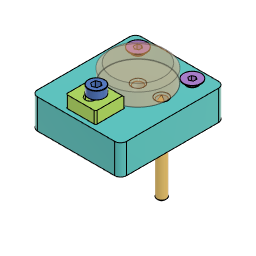
ChannelScoringJig_Parametric (Autodesk Fusion 360 design; units mm, degrees)
Autodesk Fusion 360 part; units mm, degrees
sketch "Sketch1" plane through (0, 0, 0) normal (0, 0, 1) x (1, 0, 0)
  line L0 (15, 17.5) -> (-15, 17.5)
  line L1 (-15, 17.5) -> (-15, -17.5)
  line L2 (-15, -17.5) -> (15, -17.5)
  line L3 (15, -17.5) -> (15, 17.5)
  line L4 (15, 17.5) -> (-15, -17.5) construction
  line L5 (-15, 17.5) -> (15, -17.5) construction
  dimension "d1" = 30
  dimension "d2" = 35
  constraint horizontal L0
  constraint perpendicular L0 L1
  constraint parallel L0 L2
  constraint parallel L1 L3
  constraint coincident L4 origin
  constraint coincident L5 origin
  measures "d1" distance of L0.start L0.end
  measures "d2" distance of L0.end L1.end
extrude "Extrude1" add sketch "Sketch1" along normal blind 10 makes body 1
sketch "Sketch2" plane through (0, 0, 10) normal (0, 0, 1) x (-1, 0, 0)
  line L0 (-15, 17.5) -> (-15, -17.5)
  line L1 (-15, -17.5) -> (15, -17.5)
  line L2 (15, -17.5) -> (15, 17.5)
  line L3 (15, 17.5) -> (-15, 17.5)
  circle A0 centre (9.157, -12.5) radius 1.35
  circle A1 centre (-9.157, -12.5) radius 1.35
  line L4 (9.157, -12.5) -> (-9.157, -12.5) construction
  line L5 (0, -12.5) -> (0, 0) construction
  circle A2 centre (0, -3.343) radius 12.95 construction
  line L6 (9.157, -12.5) -> (0, -3.343) construction
  line L7 (0, -3.343) -> (-9.157, -12.5) construction
  dimension "d5" = 2.7
  dimension "d42" = 5
  dimension "d67" = 25.9
  dimension "d70" = 90
  constraint coincident A0.centre L4.start
  constraint coincident A1.centre L4.end
  constraint horizontal L4
  constraint midpoint L4 L5.start
  constraint coincident L5.end origin
  constraint vertical L5
  constraint equal A0 A1
  constraint coincident L5 A2.centre
  constraint coincident A1.centre A2
  constraint coincident A2.centre L6.end
  measures "d5" diameter of A0
  measures "d42" distance of L1 L4
  measures "d67" diameter of A2
  measures "d70" angle of L6 L7
extrude "Extrude2" cut sketch "Sketch2" against normal blind 11 contours A0 | A1 bodies 1
sketch "Sketch3" plane through (0, 0, 10) normal (0, 0, 1) x (-1, 0, 0)
  line L0 (-15, 17.5) -> (-15, -17.5)
  line L1 (-15, -17.5) -> (15, -17.5)
  line L2 (15, -17.5) -> (15, 17.5)
  line L3 (15, 17.5) -> (-15, 17.5)
  circle A0 centre (0, -3.343) radius 10 construction
  circle A1 centre (9.157, -12.5) radius 2.95 construction
  circle A2 centre (0, -3.343) radius 1.6
  circle A3 centre (-8, -3.343) radius 1.6
  circle A4 centre (9.157, -12.5) radius 1.35
  point P0 (0, -13.343)
  point P1 (-10, -3.343)
  dimension "d10" = 20
  dimension "d11" = 5.9
  dimension "d12" = 3.2
  dimension "d13" = 3.2
  dimension "d53" = 2
  constraint tangent A0 A1
  constraint vertical origin A0.centre
  constraint concentric A1 A4
  constraint concentric A0 A2
  constraint coincident A0 P0
  constraint horizontal A0.centre A3.centre
  constraint coincident A0 P1
  constraint horizontal A0.centre P1
  measures "d10" diameter of A0
  measures "d11" diameter of A1
  measures "d12" diameter of A2
  measures "d13" diameter of A3
  measures "d53" distance of A3.centre P1
extrude "Extrude5" cut sketch "Sketch3" against normal blind 15 contours A2 | A3 bodies 1
sketch "Sketch6" plane through (0, 17.5, 0) normal (0, 1, 0) x (-1, 0, 0)
  line L0 (-15, 0) -> (15, 0)
  line L1 (15, 0) -> (15, 10)
  line L2 (15, 10) -> (-15, 10)
  line L3 (-15, 10) -> (-15, 0)
  line L4 (-4, 0) -> (-12, 0)
  line L5 (-12, 0) -> (-12, 3)
  line L6 (-9, 6) -> (-7, 6)
  line L7 (-4, 3) -> (-4, 0)
  arc A0 (-4, 3) -> (-7, 6) centre (-7, 3) ccw
  arc A1 (-9, 6) -> (-12, 3) centre (-9, 3) ccw
  dimension "d48" = 3
  dimension "d49" = 3
  dimension "d56" = 3
  dimension "d57" = 8
  constraint horizontal L4
  constraint vertical L5
  constraint horizontal L6
  constraint vertical L7
  constraint coincident L0 L4.start
  constraint tangent L6 A0
  constraint tangent L7 A0
  constraint tangent L5 A1
  constraint tangent L6 A1
  measures "d48" radius of A0
  measures "d49" radius of A1
  measures "d56" distance of L3 L5
  measures "d57" distance of L4.start L4.end
extrude "Extrude7" cut sketch "Sketch6" against normal blind 8.925 contours L0 L4 L5 L6 L7 A0 A1 bodies 1
sketch "Sketch10" plane through (0, 8.575, 0) normal (0, 1, 0) x (-1, 0, 0)
  arc A0 (-4, 3) -> (-7, 6) centre (-7, 3) ccw
  line L0 (-12, 0) -> (-4, 0)
  line L1 (-4, 0) -> (-4, 3)
  circle A1 centre (-8, 3) radius 1.35
  arc A2 (-9, 6) -> (-12, 3) centre (-9, 3) ccw
  line L2 (-12, 3) -> (-12, 0)
  line L3 (-7, 6) -> (-9, 6)
  dimension "d62" = 2.7
  dimension "d63" = 3
  dimension "d64" = 8
  measures "d62" diameter of A1
  measures "d63" distance of L0 A1.centre
  measures "d64" horizontal distance of origin A1.centre
extrude "Extrude10" cut sketch "Sketch10" along normal up to surface contours A1 end surface at (6.408, 3.5023, 6.6667) on bodies 1 bodies 1
fillet "Fillet2" radius 2 4 edges at (15, 17.5, 5) (-15, 17.5, 5) (15, -17.5, 5) (-15, -17.5, 5) on bodies 1
sketch "Sketch7" plane through (0, 0, 10) normal (0, 0, 1) x (-1, 0, 0)
  arc A0 (15, 15.5) -> (13, 17.5) centre (13, 15.5) ccw
  line L0 (13, 17.5) -> (-13, 17.5)
  arc A1 (-13, 17.5) -> (-15, 15.5) centre (-13, 15.5) ccw
  line L1 (-15, 15.5) -> (-15, -15.5)
  line L2 (15, -15.5) -> (15, 15.5)
  circle A2 centre (0, 10.657) radius 1.35
  circle A3 centre (0, -3.343) radius 1.6
  arc A4 (-15, -15.5) -> (-13, -17.5) centre (-13, -15.5) ccw
  line L3 (-13, -17.5) -> (13, -17.5)
  arc A5 (13, -17.5) -> (15, -15.5) centre (13, -15.5) ccw
  circle A6 centre (9.157, -12.5) radius 1.35
  circle A7 centre (-9.157, -12.5) radius 1.35
  circle A8 centre (-8, -3.343) radius 1.6
  dimension "d36" = 2.7
  dimension "d126" = 14
  constraint vertical origin A2.centre
  measures "d36" diameter of A2
  measures "d126" distance of A2.centre A3.centre
extrude "Extrude8" cut sketch "Sketch7" against normal blind 38 contours A2 bodies 1
chamfer "Chamfer1" distance 0.5 angle 45 9 edges at (9.4917, 3.9216, 0) (1.2586, -10.1689, 0) (-7.8984, 12.9882, 0) (-7.8984, 12.0118, 10) (10.4157, 12.0118, 10) (9.4917, 2.7644, 10) (1.2586, -11.1452, 10) (1.4917, 2.7644, 10) (1.4917, 3.9216, 0) on bodies 1
chamfer "Chamfer3" distance 0.5 angle 45 2 edges at (4, 13.0375, 0) (12, 13.0375, 0) measured on face at (8.4117, -8.1054, 0) measured on face at (8.4117, -8.1054, 0) on bodies 1
sketch "Sketch1 (2)" plane through (0, 0, 0) normal (0, 0, 1) x (1, 0, 0) in component "EngravingTool"
  circle A0 centre (0, 0) radius 1.5875
  dimension "d71" = 3.175
  constraint coincident A0.centre origin
  measures "d71" diameter of A0
extrude "Extrude1'" add sketch "Sketch1 (2)" against normal blind 30 separate body makes body 2 in component "EngravingTool"
chamfer "Chamfer1'" distance 1.5 angle 60 1 edges at (-1.4801, 0.5741, -30) measured on face at (-0.3879, 0.3599, -30) on bodies 2 in component "EngravingTool"
sketch "Sketch2 (2)" plane through (0, 0, -30) normal (0, 0, -1) x (1, 0, 0) in component "EngravingTool"
  circle A0 centre (0, 0) radius 0.0875
  line L0 (-4.5, 0) -> (3.5, 0)
  line L1 (3.5, 0) -> (3.5, 4)
  line L2 (3.5, 4) -> (-4.5, 4)
  line L3 (-4.5, 4) -> (-4.5, 0)
  line L4 (-4.5, 0) -> (3.5, 4) construction
  line L5 (3.5, 0) -> (-4.5, 4) construction
  point P0 (-0.5, 2)
  dimension "d76" = 8
  dimension "d77" = 4
  constraint horizontal L0
  constraint perpendicular L0 L1
  constraint parallel L0 L2
  constraint parallel L1 L3
  constraint coincident L4 P0
  constraint coincident L5 P0
  constraint coincident A0.centre L0
  measures "d76" distance of L1.end L2.end
  measures "d77" distance of L0.start L2.end
extrude "Extrude2'" cut sketch "Sketch2 (2)" against normal blind 11 contours A0 L0 | A0 L0 L1 L2 L3 picked at (0.0214, 0.0198) bodies 2 in component "EngravingTool"
fillet "Fillet1" radius 1.5875 1 edges at (0, 0, -19) on bodies 2 in component "EngravingTool"
fillet "Fillet2'" radius 0.1 1 edges at (0, 0.0875, -30) on bodies 2 in component "EngravingTool"
chamfer "Chamfer2" distance 0.5 angle 45 1 edges at (-1.4801, -0.5741, 0) measured on face at (-0.3879, 0.3599, 0) on bodies 2 in component "EngravingTool"
sketch "Sketch1 (3)" plane through (0, 0, 0) normal (0, 0, 1) x (1, 0, 0) in component "Screw1_M3 v1"
  circle A0 centre (0, 0) radius 1.5
  dimension "d760" = 3
  constraint coincident A0.centre origin
  measures "d760" diameter of A0
extrude "Extrude1''" add sketch "Sketch1 (3)" against normal blind 8 separate body makes body 3 in component "Screw1_M3 v1"
sketch "Sketch2 (3)" plane through (0, 0, -8) normal (0, 0, -1) x (1, 0, 0) in component "Screw1_M3 v1"
  circle A0 centre (0, 0) radius 1.5
  circle A1 centre (0, 0) radius 2.75
  dimension "d763" = 5.5
  constraint concentric A0 A1
  measures "d763" diameter of A1
extrude "Extrude2''" add sketch "Sketch2 (3)" along normal blind 2.75 contours A0 | A1 bodies 3 in component "Screw1_M3 v1"
sketch "Sketch3 (2)" plane through (0, 0, -10.75) normal (0, 0, -1) x (1, 0, 0) in component "Screw1_M3 v1"
  circle A0 centre (0, 0) radius 2.75
  line L0 (1.25, 0.7217) -> (0, 1.4434)
  line L1 (0, 1.4434) -> (-1.25, 0.7217)
  line L2 (-1.25, 0.7217) -> (-1.25, -0.7217)
  line L3 (-1.25, -0.7217) -> (0, -1.4434)
  line L4 (0, -1.4434) -> (1.25, -0.7217)
  line L5 (1.25, -0.7217) -> (1.25, 0.7217)
  dimension "d766" = 2.5
  constraint coincident A0.centre origin
  measures "d766" distance of L2 L5
extrude "Extrude3" cut sketch "Sketch3 (2)" against normal blind 2 contours L0 L1 L2 L3 L4 L5 bodies 3 in component "Screw1_M3 v1"
fillet "Fillet1'" radius 0.25 1 edges at (-1.3985, 0.5424, -8) on bodies 3 in component "Screw1_M3 v1"
chamfer "Chamfer1''" distance 0.1 angle 45 2 edges at (-2.5639, 0.9944, -10.75) (-2.5639, 0.9944, -8) on bodies 3 in component "Screw1_M3 v1"
chamfer "Chamfer2'" distance 0.5 angle 45 1 edges at (-1.3985, -0.5424, 0) on bodies 3 in component "Screw1_M3 v1"
sketch "Sketch1 (4)" plane through (0, 0, 0) normal (0, 0, 1) x (1, 0, 0) in component "Screw2_M3 v2"
  circle A0 centre (0, 0) radius 1.5
  dimension "d760_1" = 3
  constraint coincident A0.centre origin
  measures "d760_1" diameter of A0
extrude "Extrude1'''" add sketch "Sketch1 (4)" against normal blind 4 separate body makes body 4 in component "Screw2_M3 v2"
sketch "Sketch2 (4)" plane through (0, 0, -4) normal (0, 0, -1) x (1, 0, 0) in component "Screw2_M3 v2"
  circle A0 centre (0, 0) radius 1.5
  circle A1 centre (0, 0) radius 2.95
  dimension "d763_1" = 5.9
  constraint concentric A0 A1
  measures "d763_1" diameter of A1
extrude "Extrude2'''" add sketch "Sketch2 (4)" along normal blind 1.6 contours A0 | A1 bodies 4 in component "Screw2_M3 v2"
sketch "Sketch3 (3)" plane through (0, 0, -5.6) normal (0, 0, -1) x (1, 0, 0) in component "Screw2_M3 v2"
  circle A0 centre (0, 0) radius 2.95
  line L0 (1, 0.5774) -> (0, 1.1547)
  line L1 (0, 1.1547) -> (-1, 0.5774)
  line L2 (-1, 0.5774) -> (-1, -0.5774)
  line L3 (-1, -0.5774) -> (0, -1.1547)
  line L4 (0, -1.1547) -> (1, -0.5774)
  line L5 (1, -0.5774) -> (1, 0.5774)
  dimension "d766_1" = 2
  constraint coincident A0.centre origin
  measures "d766_1" distance of L2 L5
extrude "Extrude3'" cut sketch "Sketch3 (3)" against normal blind 1.5 contours L0 L1 L2 L3 L4 L5 bodies 4 in component "Screw2_M3 v2"
chamfer "Chamfer1'''" distance 1.4 angle 45 1 edges at (-2.7504, 1.0668, -4) on bodies 4 in component "Screw2_M3 v2"
chamfer "Chamfer2''" distance 0.3 angle 45 1 edges at (-1.3985, -0.5424, 0) on bodies 4 in component "Screw2_M3 v2"
sketch "Sketch1 (5)" plane through (0, 0, 0) normal (0, 0, 1) x (1, 0, 0) in component "Clamp"
  line L0 (5, 5) -> (-5, 5)
  line L1 (-5, 5) -> (-5, -5)
  line L2 (-5, -5) -> (5, -5)
  line L3 (5, -5) -> (5, 5)
  line L4 (5, 5) -> (-5, -5) construction
  line L5 (-5, 5) -> (5, -5) construction
  circle A0 centre (0, 11.5) radius 7.5
  line L6 (-1.7, 1.75) -> (-1.7, -1.75)
  arc A1 (-1.7, -1.75) -> (1.7, -1.75) centre (0, -1.75) ccw
  line L7 (1.7, -1.75) -> (1.7, 1.75)
  arc A2 (1.7, 1.75) -> (-1.7, 1.75) centre (0, 1.75) ccw
  line L8 (0, 1.75) -> (0, -1.75) construction
  dimension "d1_1" = 10
  dimension "d2_1" = 10
  dimension "d3_1" = 15
  dimension "d4_1" = 11.5
  dimension "d5_1" = 1.7
  dimension "d6" = 3.5
  constraint horizontal L0
  constraint perpendicular L0 L1
  constraint parallel L0 L2
  constraint parallel L1 L3
  constraint coincident L4 origin
  constraint coincident L5 origin
  constraint tangent L6 A1
  constraint tangent A1 L7
  constraint parallel L6 L7
  constraint tangent L7 A2
  constraint tangent L6 A2
  constraint perpendicular L2 L8
  constraint coincident origin L8
  constraint midpoint origin L8
  measures "d1_1" distance of L0.start L0.end
  measures "d2_1" distance of L0.start L2.end
  measures "d3_1" diameter of A0
  measures "d4_1" distance of origin A0.centre
  measures "d5_1" radius of A1
  measures "d6" distance of A2.centre A1.centre
extrude "Extrude1''''" add sketch "Sketch1 (5)" along normal blind 4 separate body contours L0 L1 L2 L3 A0 makes body 5 in component "Clamp"
chamfer "Chamfer1''''" distance 1 angle 45 2 edges at (-4.3708, 5, 4) (4.3708, 5, 4) on bodies 5 in component "Clamp"
fillet "Fillet1''" radius 0.5 4 edges at (-5, -5, 2) (5, -5, 2) (-5, 5, 1.5) (5, 5, 1.5) on bodies 5 in component "Clamp"
sketch "Sketch2 (5)" plane through (0, 0, 0) normal (0, 0, 1) x (1, 0, 0) in component "Pad"
  circle A0 centre (0, 0) radius 10
  dimension "d111" = 20
  constraint coincident A0.centre origin
  measures "d111" diameter of A0
extrude "Extrude1'''''" add sketch "Sketch2 (5)" along normal blind 6 separate body makes body 6 in component "Pad"
chamfer "Chamfer1'''''" distance 1.5 angle 45 1 edges at (-9.3233, -3.6162, 6) measured on face at (2.3712, -3.5556, 6) on bodies 6 in component "Pad"
chamfer "Chamfer2'''" distance 0.1 angle 45 1 edges at (-9.3233, -3.6162, 0) measured on face at (9.9876, -0.4985, 3) on bodies 6 in component "Pad"
component "EngravingTool" placed x (1, 0, 0) y (0, -1, 0) z (0, 0, -1) at (8, 3.343, -19.451)
component "Screw1_M3 v1" placed x (1, 0, 0) y (0, 0, 1) z (0, -1, 0) at (8, 4.45, 3)
component "Screw1_M3 v1" placed x (1, 0, 0) y (0, -1, 0) z (0, 0, -1) at (0, -10.657, 6)
component "Screw2_M3 v2" placed x (0.553608, 0.832777, 0) y (0.832777, -0.553608, 0) z (0, 0, -1) at (9.157, 12.5, 5.85)
component "Screw2_M3 v2" placed x (0.553608, 0.832777, 0) y (0.832777, -0.553608, 0) z (0, 0, -1) at (-9.157, 12.5, 5.85)
component "Clamp" placed x (1, 0, 0) y (0, 1, 0) z (0, 0, 1) at (0, -10.907, 10)
component "Pad" placed x (1, 0, 0) y (0, 1, 0) z (0, 0, 1) at (0, 3.343, 10.02)
equation "d1 = D + 10 mm"
equation "d2 = D + 15 mm"
equation "d10 = D"
equation "d11 = sd"
equation "d32 = -( D + 5.5 mm ) * 0.35"
equation "D = 20 mm" comment "Pad Diameter"
equation "d53 = b"
equation "b = 2.0 mm" comment "Channel border distance"
equation "d64 = D / 2 - b"
equation "d67 = D + sd"
equation "d71 = 0'- 1/8\""
equation "d81 = 0'- 1/16\""
equation "d763_1 = sd"
equation "sd = 5.9 mm" comment "Screw Head Diameter"
equation "d111 = D"
equation "d126 = D / 2 + 4 mm"
named bodies: "PadScribingRig", "PadScribeingClamp"
